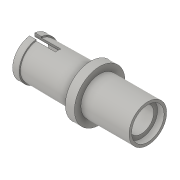
# Autodesk Inventor part: AxleNT
Saved by Autodesk Inventor 2016 (Build 200138000, 138)
## iProperties
Created: 2016-01-21
Part Number: AxleNT
Material: Generic
Document SubType Name: Modeling
Designer: 301278
Density: 1 g/cm^3
Appearance: Default
Author: 301278
Autodesk Inventor part; units mm, degrees
ref_plane "YZ Plane" through (0, 0, 0) normal (1, 0, 0) x (0, 1, 0)
ref_plane "XZ Plane" through (0, 0, 0) normal (0, 1, 0) x (-1, 0, 0)
ref_plane "XY Plane" through (0, 0, 0) normal (0, 0, 1) x (1, 0, 0)
sketch "Sketch1" plane through (0, 0, 0) normal (0, 0, 1) x (1, 0, 0)
  line L0 (0, 0) -> (0, 2.413)
  line L1 (0, 2.413) -> (8.382, 2.413)
  line L2 (8.382, 2.413) -> (8.382, 3.175)
  line L3 (8.382, 3.175) -> (9.652, 3.175)
  line L4 (9.652, 3.175) -> (9.652, 3.683)
  line L5 (9.652, 3.683) -> (0.254, 3.683)
  line L6 (0.254, 3.683) -> (0.254, 4.953)
  line L7 (0.254, 4.953) -> (-1.524, 4.953)
  line L8 (-1.524, 4.953) -> (-1.524, 3.683)
  line L9 (0, 0) -> (-1.778, 0)
  line L10 (-1.778, 0) -> (-1.778, 2.413)
  line L11 (-1.778, 2.413) -> (-6.604, 2.413)
  line L12 (-6.604, 2.413) -> (-6.604, 3.175)
  line L13 (-6.604, 3.175) -> (-12.954, 3.175)
  line L14 (-12.954, 3.175) -> (-12.954, 3.81)
  line L15 (-12.954, 3.81) -> (-11.684, 3.81)
  line L16 (-11.684, 3.81) -> (-11.684, 3.556)
  line L17 (-11.684, 3.556) -> (-1.524, 3.683)
  dimension "d0" = 2.413
  dimension "d1" = 8.382
  dimension "d2" = 0.762
  dimension "d3" = 1.27
  dimension "d4" = 0.508
  dimension "d5" = 9.398
  dimension "d6" = 1.27
  dimension "d7" = 1.778
  dimension "d8" = 1.27
  dimension "d9" = 1.778
  dimension "d10" = 2.413
  dimension "d11" = 4.826
  dimension "d12" = 0.762
  dimension "d13" = 6.35
  dimension "d14" = 0.635
  dimension "d15" = 1.27
  dimension "d16" = 0.254
  constraints: 36 end point, 9 perpendicular, 4 horizontal, 2 vertical, 1 parallel, 1 point on line
  measures "d0" distance of L0.start L0.end
  measures "d1" distance of L0.end L1.end
  measures "d2" distance of L1.end L2.end
  measures "d3" distance of L2.end L3.end
  measures "d4" distance of L3.end L4.end
  measures "d5" distance of L4.end L5.end
  measures "d6" distance of L5.end L6.end
  measures "d7" distance of L6.end L7.end
  measures "d8" distance of L7.end L8.end
  measures "d9" distance of L0.start L9.end
  measures "d10" distance of L9.end L10.end
  measures "d11" distance of L10.end L11.end
  measures "d12" distance of L11.end L12.end
  measures "d13" distance of L12.end L13.end
  measures "d14" distance of L13.end L14.end
  measures "d15" distance of L14.end L15.end
  measures "d16" distance of L15.end L16.end
revolve "Revolution1" add sketch "Sketch1" angle 360 about axis through (0, 0, 0) along (-1, 0, 0)
sketch "Sketch2" plane through (-12.954, 0, 0) normal (-1, 0, 0) x (0, 0, 1)
  circle A0 centre (0, 0) radius 3.81 projected
  line L0 (-0.508, 4.1374) -> (0.508, 4.1374)
  line L1 (0.508, 4.1374) -> (0.508, -4.4161)
  line L2 (0.508, -4.4161) -> (-0.508, -4.4161)
  line L3 (-0.508, -4.4161) -> (-0.508, 4.1374)
  dimension "d18" = 1.016
  constraints: 8 end point, 2 parallel, 1 horizontal, 1 perpendicular
  measures "d18" distance of L1.end L2.end
extrude "Extrusion1" cut sketch "Sketch2" against normal blind 5.08 contours L1 A0 L3 | A0 L3 L0 L1 | L1 L2 L3 A0
body "Solid1"
